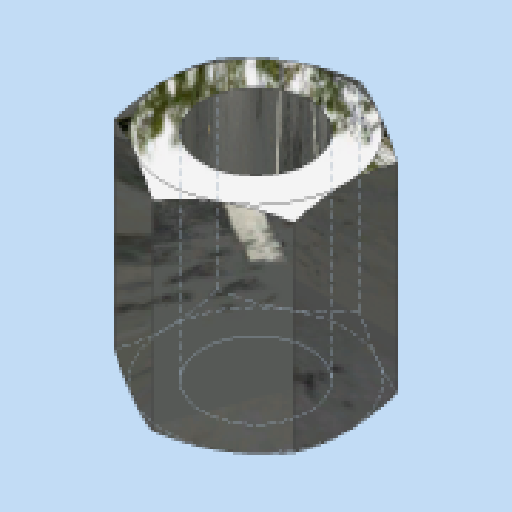
# Autodesk Inventor part: M3_H8.0mm_board_spacer
Saved by Autodesk Inventor 2024 (Build 280153000, 153)
## iProperties
Created: 2025-05-08
Part Number: M3_H8.0mm_board_spacer
Material: Nickel-Copper Alloy 400
Document SubType Name: Modeling
Designer: XxPan
Density: 8.83 g/cm^3
Appearance: Chrome - Polished
Author: XxPan
Autodesk Inventor part; units mm, degrees
ref_plane "YZ Plane" through (0, 0, 0) normal (1, 0, 0) x (0, 1, 0)
ref_plane "XZ Plane" through (0, 0, 0) normal (0, 1, 0) x (-1, 0, 0)
ref_plane "XY Plane" through (0, 0, 0) normal (0, 0, 1) x (1, 0, 0)
sketch "Sketch1" plane through (0, 0, 0) normal (0, 1, 0) x (-1, 0, 0)
  line L0 (0, -2.8868) -> (-2.5, -1.4434)
  line L1 (-2.5, -1.4434) -> (-2.5, 1.4434)
  line L2 (-2.5, 1.4434) -> (0, 2.8868)
  line L3 (0, 2.8868) -> (2.5, 1.4434)
  line L4 (2.5, 1.4434) -> (2.5, -1.4434)
  line L5 (2.5, -1.4434) -> (0, -2.8868)
  point P0 (0, 0)
  point P1 (0, 0)
  dimension "d0" = 5
  constraints: 12 end point, 1 coincident, 13 other
  measures "d0" distance between parallel lines of L1 L4
extrude "Extrusion1" add sketch "Sketch1" along normal blind 6
sketch "Sketch2" plane through (0, 6, 0) normal (0, 1, 0) x (1, 0, 0)
  point P0 (0, 0)
  point P1 (0, 0)
  constraints: 1 coincident
hole "Hole1" at (0, 6, 0) direction (0, -1, 0) diameter 3 end through all
sketch "Sketch3" plane through (0, 0, 0) normal (0, 0, 1) x (1, 0, 0)
  line L0 (0, 6) -> (2.5, 6) projected
  line L1 (2.5, 6) -> (4.5, 6)
  line L2 (2.5, 6) -> (4.5, 4.8453)
  line L3 (2.5, 6) -> (4.8094, 6) construction
  line L4 (4.5, 4.8453) -> (4.5, 6)
  line L5 (2.5, 0) -> (2.5, 6) projected
  line L6 (2.5, 0) -> (4.5, 0)
  line L7 (2.5, 0) -> (4.5, 1.1547)
  line L8 (2.5, 0) -> (4.8094, 0) construction
  line L9 (4.5, 1.1547) -> (4.5, 0)
  line L10 (0, -1.6) -> (0, 9.6) projected
  point P0 (0, 0)
  dimension "d10" = 30
  dimension "d11" = 2
  dimension "d12" = 30
  constraints: 16 end point, 4 horizontal, 2 equal length, 2 vertical, 1 collinear
  measures "d10" angle of L2 L3
  measures "d11" distance of L0.end L1.end
  measures "d12" angle of L8 L7
revolve "Revolution1" cut sketch "Sketch3" angle 360 about axis through (0, -10, 0) along (0, 1, 0)
body "Solid1"
